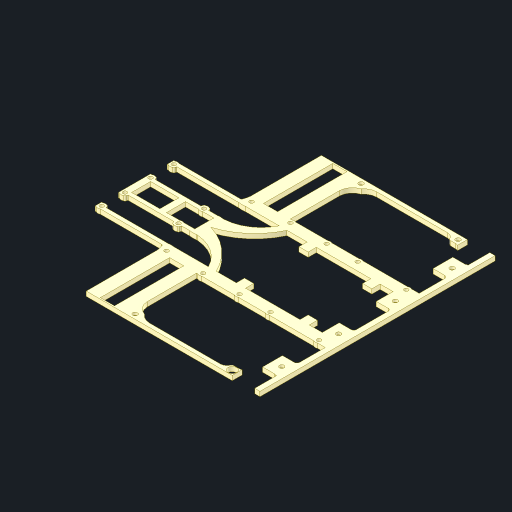
# Autodesk Inventor part: base
Saved by Autodesk Inventor 2023 (Build 270158000, 158)
## iProperties
Created: 2024-05-25
Part Number: base
Material: Nylon 6
Document SubType Name: Modeling
Designer: szymo
Density: 1.12 g/cm^3
Appearance: Nylon 6
Mass: 126.189 g
Surface Area: 671.47 cm^2
Volume: 112.669 cm^3
Author: szymo
Autodesk Inventor part; units mm, degrees
ref_plane "YZ Plane" through (0, 0, 0) normal (1, 0, 0) x (0, 1, 0)
ref_plane "XZ Plane" through (0, 0, 0) normal (0, 1, 0) x (-1, 0, 0)
ref_plane "XY Plane" through (0, 0, 0) normal (0, 0, 1) x (1, 0, 0)
sketch "Sketch1" plane through (0, 0, 0) normal (0, 1, 0) x (-1, 0, 0)
  line L0 (99, 89) -> (-99, 89)
  line L1 (-99, 89) -> (-99, -89)
  line L2 (-99, -89) -> (99, -89)
  line L3 (99, -89) -> (99, 89)
  line L4 (99, 89) -> (-99, -89) construction
  line L5 (-99, 89) -> (99, -89) construction
  line L6 (-85, 89) -> (-85, -89)
  line L7 (-64, 89) -> (-64, 72.5)
  line L8 (-64, 72.5) -> (-81, 72.5)
  line L9 (-81, -72.5) -> (-64, -72.5)
  line L10 (-64, -72.5) -> (-64, -89)
  line L11 (-81, -89) -> (-81, 89)
  point P0 (0, 0)
  dimension "d0" = 198
  dimension "d1" = 178
  dimension "d2" = 14
  dimension "d3" = 16.5
  dimension "d4" = 16.5
  dimension "d9" = 4
  dimension "d10" = 17
  dimension "d11" = 17
  constraints: 24 end point, 8 point on line, 6 perpendicular, 2 horizontal, 2 midpoint, 2 parallel, 1 vertical
  measures "d0" distance of L2.end L1.end
  measures "d1" distance of L1.end L0.end
  measures "d2" distance between parallel lines of L6 L1
  measures "d3" distance between parallel lines of L0 L8
  measures "d4" distance between parallel lines of L9 L2
  measures "d9" distance between parallel lines of L11 L6
  measures "d10" distance between parallel lines of L10 L11
  measures "d11" distance between parallel lines of L11 L7
extrude "Extrusion1" add sketch "Sketch1" along normal blind 3.5 contours L3 L2 L10 L9 L11 L8 L7 L0 | L11 L2 L6 L0
sketch "Sketch2" plane through (0, 0, 0) normal (0, -1, 0) x (1, 0, 0)
  circle A0 centre (77, -64.5) radius 1.2295
  circle A1 centre (77, -21.5) radius 1.2295
  circle A2 centre (77, 21.5) radius 1.2295
  circle A3 centre (77, 64.5) radius 1.2295
  arc A4 (56.6186, 83.1429) -> (58.4256, 82) centre (58.4256, 84) ccw
  line L0 (62, 82) -> (58.4256, 82)
  arc A5 (66.9487, 77.7143) -> (62, 82) centre (62, 77) ccw
  arc A6 (66.9487, 77.7143) -> (68.9282, 76) centre (68.9282, 78) ccw
  line L1 (72.3229, 76) -> (68.9282, 76)
  arc A7 (72.3229, 76) -> (74.3229, 78) centre (72.3229, 78) ccw
  line L2 (74.3229, 81.0104) -> (74.3229, 78)
  arc A8 (79, 86) -> (74.3229, 81.0104) centre (79.3229, 81.0104) ccw
  line L3 (79, 89) -> (79, 86)
  line L4 (-46.5, 89) -> (79, 89)
  line L5 (-46.5, 89) -> (-46.5, 73)
  line L6 (-39.246, 73) -> (-46.5, 73)
  spline S0 degree 3 poles (-38.725, 73.0306) (-38.9029, 73.01) (-39.0786, 73) (-39.246, 73) knots 0 0 0 0 1 1 1 1
  line L7 (-38.725, 88) -> (-38.725, 73.0306)
  line L8 (-24.275, 88) -> (-38.725, 88)
  line L9 (-24.275, 73.0306) -> (-24.275, 88)
  spline S1 degree 3 poles (-23.754, 73) (-23.9214, 73) (-24.0971, 73.01) (-24.275, 73.0306) knots 0 0 0 0 1 1 1 1
  line L10 (-16.5, 73) -> (-23.754, 73)
  arc A9 (-9.5, 82) -> (-16.5, 73) centre (-6.5148, 72.456) ccw
  arc A10 (-1.5, 86) -> (-9.5, 82) centre (-1.5, 76) ccw
  line L11 (52.101, 86) -> (-1.5, 86)
  arc A11 (56.6186, 83.1429) -> (52.101, 86) centre (52.101, 81) ccw
  circle A12 centre (70, 79.5) radius 1.75
  circle A13 centre (-13, 85.5) radius 2.3
  circle A14 centre (60.5017, 85.4375) radius 2.3
  circle A15 centre (70, -82.5) radius 1.75
  arc A16 (58.4256, -82) -> (56.6186, -83.1429) centre (58.4256, -84) ccw
  arc A17 (52.101, -86) -> (56.6186, -83.1429) centre (52.101, -81) ccw
  line L12 (52.101, -86) -> (-1.5, -86)
  arc A18 (-9.5, -82) -> (-1.5, -86) centre (-1.5, -76) ccw
  arc A19 (-16.5, -73) -> (-9.5, -82) centre (-6.5148, -72.456) ccw
  line L13 (-16.5, -73) -> (-23.754, -73)
  spline S2 degree 3 poles (-23.754, -73) (-23.9214, -73) (-24.0971, -73.01) (-24.275, -73.0306) knots 0 0 0 0 1 1 1 1
  line L14 (-24.275, -73.0306) -> (-24.275, -88)
  line L15 (-24.275, -88) -> (-38.725, -88)
  line L16 (-38.725, -88) -> (-38.725, -73.0306)
  spline S3 degree 3 poles (-38.725, -73.0306) (-38.9029, -73.01) (-39.0786, -73) (-39.246, -73) knots 0 0 0 0 1 1 1 1
  line L17 (-39.246, -73) -> (-46.5, -73)
  line L18 (-46.5, -89) -> (-46.5, -73)
  line L19 (-46.5, -89) -> (79, -89)
  line L20 (79, -89) -> (79, -86)
  arc A20 (74.3229, -81.0104) -> (79, -86) centre (79.3229, -81.0104) ccw
  line L21 (74.3229, -81.0104) -> (74.3229, -78)
  arc A21 (74.3229, -78) -> (72.3229, -76) centre (72.3229, -78) ccw
  line L22 (72.3229, -76) -> (68.9282, -76)
  arc A22 (68.9282, -76) -> (66.9487, -77.7143) centre (68.9282, -78) ccw
  arc A23 (62, -82) -> (66.9487, -77.7143) centre (62, -77) ccw
  line L23 (62, -82) -> (58.4256, -82)
  circle A24 centre (-13, -85.5) radius 2.3
  circle A25 centre (60.5017, -85.4375) radius 2.3
  point P0 (0, 0)
  point P1 (-13, -85.5)
  point P2 (-13, 85.5)
  constraints: 6 coincident
hole "m3" at (-13, 0, -85.5) at (60.5017, 0, -85.4375) at (-13, 0, 85.5) at (60.5017, 0, 85.4375) at (77, 0, 64.5) at (77, 0, 21.5) at (77, 0, -21.5) at (77, 0, -64.5) direction (0, 1, 0) diameter 3.6 end through all countersink diameter 6.7 countersink angle 90 clearance for "Countersunk Flat Head Screw ISO 2009/7046" size "M3" standard "ISO"
sketch "Sketch3" plane through (0, 0, 0) normal (0, -1, 0) x (1, 0, 0)
  circle A0 centre (-96.5, -27.3) radius 1.75
  circle A1 centre (-96.5, -9.7) radius 1.75
  circle A2 centre (-96.5, 9.7) radius 1.75
  circle A3 centre (-96.5, 27.3) radius 1.75
  circle A4 centre (-56, 9.7) radius 1.75
  circle A5 centre (-56, -9.7) radius 1.75
  circle A6 centre (-42.5596, -32.1689) radius 1.5
  circle A7 centre (-42.5596, 32.1689) radius 1.75
  circle A8 centre (-13.9698, 33) radius 1.75
  circle A9 centre (13.5198, 33) radius 1.75
  circle A10 centre (37.0073, 33) radius 1.75
  circle A11 centre (73.7355, 33) radius 1.75
  circle A12 centre (73.7355, -33) radius 1.75
  circle A13 centre (37.0073, -33) radius 1.75
  circle A14 centre (-96.5, -27.3) radius 1.75
  circle A15 centre (73.7355, -33) radius 1.75
  circle A16 centre (13.5198, -33) radius 1.75
  circle A17 centre (-42.5596, -32.1689) radius 1.75
  circle A18 centre (-13.9698, -33) radius 1.75
  arc A19 (-94, -25.8) -> (-95, -24.8) centre (-95, -25.8) ccw
  line L0 (-95, -24.8) -> (-99, -24.8)
  line L1 (-99, -29.8) -> (-99, -24.8)
  line L2 (-48.6566, -29.8) -> (-99, -29.8)
  arc A20 (-47.7313, -30.4207) -> (-48.6566, -29.8) centre (-48.6566, -30.8) ccw
  arc A21 (-46.5, -35.5) -> (-47.7313, -30.4207) centre (-63.78, -37) ccw
  line L3 (79, -35.5) -> (-46.5, -35.5)
  line L4 (79, -35.5) -> (79, -30.5)
  line L5 (79, -30.5) -> (-33.3917, -30.5)
  arc A22 (-40.5373, -26.8) -> (-33.3917, -30.5) centre (-33.3917, -21.75) ccw
  line L6 (-40.5373, -26.8) -> (-41.9987, -26.8)
  spline S0 degree 3 poles (-46.8237, -26.8) (-46.5789, -26.8) (-46.2862, -26.7761) (-45.5332, -26.6913) (-44.9243, -26.6) (-44.4112, -26.6) (-43.8981, -26.6) (-43.2892, -26.6913) (-42.5362, -26.7761) (-42.2435, -26.8) (-41.9987, -26.8) knots 0 0 0 0 0.161475 0.161475 0.5 0.5 0.5 0.838525 0.838525 1 1 1 1
  line L7 (-46.8237, -26.8) -> (-94, -26.8)
  line L8 (-94, -26.8) -> (-94, -25.8)
  line L9 (28.681, 30.5) -> (45.3337, 30.5)
  circle A23 centre (37.0073, 33) radius 1.75
  circle A24 centre (-96.5, 27.3) radius 1.75
  circle A25 centre (73.7355, 33) radius 1.75
  circle A26 centre (13.5198, 33) radius 1.75
  circle A27 centre (-42.5596, 32.1689) radius 1.75
  circle A28 centre (-13.9698, 33) radius 1.75
  arc A29 (-95, 24.8) -> (-94, 25.8) centre (-95, 25.8) ccw
  line L10 (-94, 26.8) -> (-94, 25.8)
  line L11 (-46.8237, 26.8) -> (-94, 26.8)
  spline S1 degree 3 poles (-46.8237, 26.8) (-46.5789, 26.8) (-46.2862, 26.7761) (-45.5332, 26.6913) (-44.9243, 26.6) (-44.4112, 26.6) (-43.8981, 26.6) (-43.2892, 26.6913) (-42.5362, 26.7761) (-42.2435, 26.8) (-41.9987, 26.8) knots 0 0 0 0 0.161475 0.161475 0.5 0.5 0.5 0.838525 0.838525 1 1 1 1
  line L12 (-40.5373, 26.8) -> (-41.9987, 26.8)
  arc A30 (-33.3917, 30.5) -> (-40.5373, 26.8) centre (-33.3917, 21.75) ccw
  line L13 (79, 30.5) -> (-33.3917, 30.5)
  line L14 (79, 35.5) -> (79, 30.5)
  line L15 (79, 35.5) -> (-46.5, 35.5)
  arc A31 (-47.7313, 30.4207) -> (-46.5, 35.5) centre (-63.78, 37) ccw
  arc A32 (-48.6566, 29.8) -> (-47.7313, 30.4207) centre (-48.6566, 30.8) ccw
  line L16 (-48.6566, 29.8) -> (-99, 29.8)
  line L17 (-99, 29.8) -> (-99, 24.8)
  line L18 (-95, 24.8) -> (-99, 24.8)
  point P0 (0, 0)
  constraints: 16 coincident
hole "m2.5" at (73.7355, 0, -33) at (37.0073, 0, -33) at (13.5198, 0, -33) at (-13.9698, 0, -33) at (-42.5596, 0, -32.1689) at (73.7355, 0, 33) at (37.0073, 0, 33) at (13.5198, 0, 33) at (-13.9698, 0, 33) at (-42.5596, 0, 32.1689) at (-56, 0, 9.7) at (-56, 0, -9.7) at (-96.5, 0, -9.7) at (-96.5, 0, 9.7) at (-96.5, 0, 27.3) at (-96.5, 0, -27.3) direction (0, 1, 0) diameter 3.1 end through all countersink diameter 5.8 countersink angle 90 clearance for "Countersunk Flat Head Screw ISO 2009/7046" size "M2.5" standard "ISO"
sketch "Sketch4" plane through (0, 0, 0) normal (0, 1, 0) x (1, 0, 0)
  line L0 (-36.8852, -40.5) -> (-31.5, -40.5)
  line L1 (-31.5, -40.5) -> (-26.1148, -40.5)
  line L2 (-26.1148, -40.5) -> (-26.1148, -68.2)
  line L3 (-26.1148, -68.2) -> (-36.8852, -68.2)
  line L4 (-36.8852, -68.2) -> (-36.8852, -40.5)
  line L5 (-26.1148, 40.5) -> (-31.5, 40.5)
  line L6 (-31.5, 40.5) -> (-36.8852, 40.5)
  line L7 (-36.8852, 40.5) -> (-36.8852, 68.2)
  line L8 (-36.8852, 68.2) -> (-26.1148, 68.2)
  line L9 (-26.1148, 68.2) -> (-26.1148, 40.5)
  line L10 (-24.275, 88) -> (-38.725, 88)
  line L11 (-46.5, 89) -> (-46.5, 73)
  line L12 (-46.5, 89) -> (79, 89)
  line L13 (79, 89) -> (79, 86)
  line L14 (74.3229, 81.0104) -> (74.3229, 78)
  line L15 (74.3229, -81.0104) -> (74.3229, -78)
  line L16 (79, -89) -> (79, -86)
  line L17 (-46.5, -89) -> (79, -89)
  line L18 (-46.5, -89) -> (-46.5, -73)
  circle A0 centre (70, -79.5) radius 1.75
  circle A1 centre (37.0073, 33) radius 1.75
  circle A2 centre (-96.5, 27.3) radius 1.75
  circle A3 centre (73.7355, 33) radius 1.75
  circle A4 centre (13.5198, 33) radius 1.75
  circle A5 centre (-42.5596, 32.1689) radius 1.75
  circle A6 centre (-13.9698, 33) radius 1.75
  arc A7 (-95, 24.8) -> (-94, 25.8) centre (-95, 25.8) ccw
  line L19 (-95, 24.8) -> (-99, 24.8)
  line L20 (-99, 29.8) -> (-99, 24.8)
  line L21 (-48.6566, 29.8) -> (-99, 29.8)
  arc A8 (-48.6566, 29.8) -> (-47.7313, 30.4207) centre (-48.6566, 30.8) ccw
  arc A9 (-47.7313, 30.4207) -> (-46.5, 35.5) centre (-63.78, 37) ccw
  line L22 (79, 35.5) -> (-46.5, 35.5)
  line L23 (79, 35.5) -> (79, 30.5)
  line L24 (79, 30.5) -> (-33.3917, 30.5)
  arc A10 (-33.3917, 30.5) -> (-40.5373, 26.8) centre (-33.3917, 21.75) ccw
  line L25 (-40.5373, 26.8) -> (-41.9987, 26.8)
  spline S0 degree 3 poles (-46.8237, 26.8) (-46.5789, 26.8) (-46.2862, 26.7761) (-45.5332, 26.6913) (-44.9243, 26.6) (-44.4112, 26.6) (-43.8981, 26.6) (-43.2892, 26.6913) (-42.5362, 26.7761) (-42.2435, 26.8) (-41.9987, 26.8) knots 0 0 0 0 0.161475 0.161475 0.5 0.5 0.5 0.838525 0.838525 1 1 1 1
  line L26 (-46.8237, 26.8) -> (-94, 26.8)
  line L27 (-94, 26.8) -> (-94, 25.8)
  circle A11 centre (37.0073, -33) radius 1.75
  circle A12 centre (-96.5, -27.3) radius 1.75
  circle A13 centre (73.7355, -33) radius 1.75
  circle A14 centre (13.5198, -33) radius 1.75
  circle A15 centre (-42.5596, -32.1689) radius 1.75
  circle A16 centre (-13.9698, -33) radius 1.75
  arc A17 (-94, -25.8) -> (-95, -24.8) centre (-95, -25.8) ccw
  line L28 (-94, -26.8) -> (-94, -25.8)
  line L29 (-46.8237, -26.8) -> (-94, -26.8)
  spline S1 degree 3 poles (-46.8237, -26.8) (-46.5789, -26.8) (-46.2862, -26.7761) (-45.5332, -26.6913) (-44.9243, -26.6) (-44.4112, -26.6) (-43.8981, -26.6) (-43.2892, -26.6913) (-42.5362, -26.7761) (-42.2435, -26.8) (-41.9987, -26.8) knots 0 0 0 0 0.161475 0.161475 0.5 0.5 0.5 0.838525 0.838525 1 1 1 1
  line L30 (-40.5373, -26.8) -> (-41.9987, -26.8)
  arc A18 (-40.5373, -26.8) -> (-33.3917, -30.5) centre (-33.3917, -21.75) ccw
  line L31 (79, -30.5) -> (-33.3917, -30.5)
  line L32 (79, -35.5) -> (79, -30.5)
  line L33 (79, -35.5) -> (-46.5, -35.5)
  arc A19 (-46.5, -35.5) -> (-47.7313, -30.4207) centre (-63.78, -37) ccw
  arc A20 (-47.7313, -30.4207) -> (-48.6566, -29.8) centre (-48.6566, -30.8) ccw
  line L34 (-48.6566, -29.8) -> (-99, -29.8)
  line L35 (-99, -29.8) -> (-99, -24.8)
  line L36 (-95, -24.8) -> (-99, -24.8)
  line L37 (44.7969, 39.7458) -> (-15.2031, 39.7458) construction
  line L38 (-15.2031, 39.7458) -> (-15.2031, 69.7458) construction
  line L39 (44.7969, 69.7458) -> (-15.2031, 69.7458) construction
  line L40 (44.7969, 39.7458) -> (44.7969, 69.7458) construction
  line L41 (44.5627, -68.989) -> (-15.4373, -68.989) construction
  line L42 (-15.4373, -68.989) -> (-15.4373, -38.989) construction
  line L43 (44.5627, -38.989) -> (-15.4373, -38.989) construction
  line L44 (44.5627, -68.989) -> (44.5627, -38.989) construction
  line L45 (85, 89) -> (99, 89)
  line L46 (99, 89) -> (99, -89)
  line L47 (85, -89) -> (99, -89)
  line L48 (85, 89) -> (85, -89)
  circle A21 centre (77, -21.5) radius 1.2295
  circle A22 centre (77, 64.5) radius 1.2295
  circle A23 centre (77, 21.5) radius 1.2295
  circle A24 centre (77, -64.5) radius 1.2295
  line L49 (70, 72) -> (79, 72)
  arc A25 (79, 72) -> (81, 74) centre (79, 74) ccw
  line L50 (81, 74) -> (81, 89)
  line L51 (81, 89) -> (85, 89)
  line L52 (85, 89) -> (85, -89)
  line L53 (81, -89) -> (85, -89)
  line L54 (81, -89) -> (81, -74)
  arc A26 (81, -74) -> (79, -72) centre (79, -74) ccw
  line L55 (79, -72) -> (70, -72)
  line L56 (70, -57) -> (70, -72)
  line L57 (70, -57) -> (79, -57)
  arc A27 (79, -57) -> (81, -55) centre (79, -55) ccw
  line L58 (81, -55) -> (81, -31)
  arc A28 (81, -31) -> (79, -29) centre (79, -31) ccw
  line L59 (79, -29) -> (70, -29)
  line L60 (70, -14) -> (70, -29)
  line L61 (70, -14) -> (79, -14)
  arc A29 (79, -14) -> (81, -12) centre (79, -12) ccw
  line L62 (81, -12) -> (81, 12)
  arc A30 (81, 12) -> (79, 14) centre (79, 12) ccw
  line L63 (79, 14) -> (70, 14)
  line L64 (70, 29) -> (70, 14)
  line L65 (70, 29) -> (79, 29)
  arc A31 (79, 29) -> (81, 31) centre (79, 31) ccw
  line L66 (81, 31) -> (81, 55)
  arc A32 (81, 55) -> (79, 57) centre (79, 55) ccw
  line L67 (79, 57) -> (70, 57)
  line L68 (70, 72) -> (70, 57)
  line L69 (60, -27.5) -> (5, -27.5)
  line L70 (5, -27.5) -> (5, 27.5)
  line L71 (5, 27.5) -> (60, 27.5)
  line L72 (60, 27.5) -> (60, -27.5)
  circle A33 centre (56.6, -24.1) radius 1.6
  circle A34 centre (8.4, -24.1) radius 1.6
  circle A35 centre (56.6, 24.1) radius 1.6
  circle A36 centre (8.4, 24.1) radius 1.6
  line L73 (-99, -7) -> (-37.5, -7) construction
  line L74 (-99, 7) -> (-99, -7) construction
  line L75 (-37.5, 7) -> (-99, 7) construction
  line L76 (-37.5, -7) -> (-37.5, 7) construction
  circle A37 centre (-56, 9.7) radius 1.75
  circle A38 centre (-96.5, 9.7) radius 1.75
  arc A39 (-57.5, 12.2) -> (-58.5, 11.2) centre (-57.5, 11.2) ccw
  line L77 (-57.5, 12.2) -> (-54.5, 12.2)
  arc A40 (-53.5, 11.2) -> (-54.5, 12.2) centre (-54.5, 11.2) ccw
  line L78 (-53.5, 11.2) -> (-53.5, 10.2)
  line L79 (-53.5, 10.2) -> (-46.8237, 10.2)
  spline S2 degree 3 poles (-41.9987, 10.2) (-42.2435, 10.2) (-42.5362, 10.2239) (-43.2892, 10.3087) (-43.8981, 10.4) (-44.4112, 10.4) (-44.9243, 10.4) (-45.5332, 10.3087) (-46.2862, 10.2239) (-46.5789, 10.2) (-46.8237, 10.2) knots 0 0 0 0 0.161475 0.161475 0.5 0.5 0.5 0.838525 0.838525 1 1 1 1
  line L80 (-41.9987, 10.2) -> (-41.148, 10.2)
  line L81 (-41.148, 10.2) -> (-41.148, 7.2)
  line L82 (-41.148, 7.2) -> (-99, 7.2)
  line L83 (-99, 7.2) -> (-99, 12.2)
  line L84 (-99, 12.2) -> (-95, 12.2)
  arc A41 (-94, 11.2) -> (-95, 12.2) centre (-95, 11.2) ccw
  line L85 (-94, 10.2) -> (-94, 11.2)
  line L86 (-94, 10.2) -> (-58.5, 10.2)
  line L87 (-58.5, 10.2) -> (-58.5, 11.2)
  circle A42 centre (-56, -9.7) radius 1.75
  circle A43 centre (-96.5, -9.7) radius 1.75
  arc A44 (-58.5, -11.2) -> (-57.5, -12.2) centre (-57.5, -11.2) ccw
  line L88 (-58.5, -10.2) -> (-58.5, -11.2)
  line L89 (-94, -10.2) -> (-58.5, -10.2)
  line L90 (-94, -10.2) -> (-94, -11.2)
  arc A45 (-95, -12.2) -> (-94, -11.2) centre (-95, -11.2) ccw
  line L91 (-99, -12.2) -> (-95, -12.2)
  line L92 (-99, -7.2) -> (-99, -12.2)
  line L93 (-41.148, -7.2) -> (-99, -7.2)
  line L94 (-41.148, -10.2) -> (-41.148, -7.2)
  line L95 (-41.9987, -10.2) -> (-41.148, -10.2)
  spline S3 degree 3 poles (-41.9987, -10.2) (-42.2435, -10.2) (-42.5362, -10.2239) (-43.2892, -10.3087) (-43.8981, -10.4) (-44.4112, -10.4) (-44.9243, -10.4) (-45.5332, -10.3087) (-46.2862, -10.2239) (-46.5789, -10.2) (-46.8237, -10.2) knots 0 0 0 0 0.161475 0.161475 0.5 0.5 0.5 0.838525 0.838525 1 1 1 1
  line L96 (-53.5, -10.2) -> (-46.8237, -10.2)
  line L97 (-53.5, -11.2) -> (-53.5, -10.2)
  arc A46 (-54.5, -12.2) -> (-53.5, -11.2) centre (-54.5, -11.2) ccw
  line L98 (-57.5, -12.2) -> (-54.5, -12.2)
  line L99 (81, 35.5) -> (-46.5, 35.5)
  line L100 (-46.5, 35.5) -> (-46.5, 29.8)
  line L101 (-46.5, 29.8) -> (-99, 29.8)
  line L102 (-99, 29.8) -> (-99, 24.8)
  line L103 (-99, 24.8) -> (-95, 24.8)
  line L104 (-94, 25.8) -> (-94, 26.8)
  line L105 (-94, 26.8) -> (-40.5373, 26.8)
  line L106 (-40.5373, 26.8) -> (70, 26.8)
  line L107 (81, -35.5) -> (-46.5, -35.5)
  line L108 (-46.5, -35.5) -> (-46.5, -29.8)
  line L109 (-46.5, -29.8) -> (-99, -29.8)
  line L110 (-99, -24.8) -> (-99, -29.8)
  line L111 (-99, -24.8) -> (-95, -24.8)
  line L112 (-94, -25.8) -> (-94, -26.8)
  line L113 (-94, -26.8) -> (-40.5373, -26.8)
  line L114 (-40.5373, -26.8) -> (70, -26.8)
  line L115 (60.1, 27.6) -> (53.1, 27.6)
  line L116 (53.1, 27.6) -> (53.1, 20.6)
  line L117 (53.1, 20.6) -> (60.1, 20.6)
  line L118 (60.1, 20.6) -> (60.1, 27.6)
  line L119 (60.1, 27.6) -> (53.1, 20.6) construction
  line L120 (53.1, 27.6) -> (60.1, 20.6) construction
  line L121 (60.1, -20.6) -> (53.1, -20.6)
  line L122 (53.1, -20.6) -> (53.1, -27.6)
  line L123 (53.1, -27.6) -> (60.1, -27.6)
  line L124 (60.1, -27.6) -> (60.1, -20.6)
  line L125 (60.1, -20.6) -> (53.1, -27.6) construction
  line L126 (53.1, -20.6) -> (60.1, -27.6) construction
  line L127 (11.9, -20.6) -> (4.9, -20.6)
  line L128 (4.9, -20.6) -> (4.9, -27.6)
  line L129 (4.9, -27.6) -> (11.9, -27.6)
  line L130 (11.9, -27.6) -> (11.9, -20.6)
  line L131 (11.9, -20.6) -> (4.9, -27.6) construction
  line L132 (4.9, -20.6) -> (11.9, -27.6) construction
  line L133 (11.9, 27.6) -> (4.9, 27.6)
  line L134 (4.9, 27.6) -> (4.9, 20.6)
  line L135 (4.9, 20.6) -> (11.9, 20.6)
  line L136 (11.9, 20.6) -> (11.9, 27.6)
  line L137 (11.9, 27.6) -> (4.9, 20.6) construction
  line L138 (4.9, 27.6) -> (11.9, 20.6) construction
  line L139 (-99, 7.2) -> (-94, 7.2)
  line L140 (-94, 7.2) -> (-94, -7.2)
  line L141 (-94, -7.2) -> (-99, -7.2)
  line L142 (-99, -7.2) -> (-99, 7.2)
  line L143 (-41.148, 7.2) -> (-46.148, 7.2)
  line L144 (-46.148, 7.2) -> (-46.148, -7.2)
  line L145 (-46.148, -7.2) -> (-41.148, -7.2)
  line L146 (-41.148, -7.2) -> (-41.148, 7.2)
  line L147 (-72.574, 7.2) -> (-67.574, 7.2)
  line L148 (-67.574, 7.2) -> (-67.574, -7.2)
  line L149 (-67.574, -7.2) -> (-72.574, -7.2)
  line L150 (-72.574, -7.2) -> (-72.574, 7.2)
  arc A47 (-41.148, 10.2) -> (-13.9698, 33) centre (-43.1088, 40.1359) ccw
  arc A48 (-13.9698, -33) -> (-41.148, -10.2) centre (-43.1088, -40.1359) ccw
  line L151 (-13.9698, 33) -> (-7.9698, 33)
  line L152 (-13.9698, -33) -> (-7.9698, -33)
  arc A49 (-41.148, 0) -> (-7.9698, 33) centre (-55.7201, 47.8294) ccw
  arc A50 (-7.9698, -33) -> (-41.148, 0) centre (-55.7201, -47.8294) ccw
  line L153 (-36.8852, 35.5) -> (-46.5, 35.5)
  line L154 (-46.5, 35.5) -> (-46.5, 89)
  line L155 (-46.5, 89) -> (-36.8852, 89)
  line L156 (-36.8852, 89) -> (-36.8852, 35.5)
  line L157 (-26.1148, 35.5) -> (-16.5, 35.5)
  line L158 (-16.5, 35.5) -> (-16.5, 89)
  line L159 (-16.5, 89) -> (-26.1148, 89)
  line L160 (-26.1148, 89) -> (-26.1148, 35.5)
  line L161 (-46.5, -35.5) -> (-36.8852, -35.5)
  line L162 (-36.8852, -35.5) -> (-36.8852, -89)
  line L163 (-36.8852, -89) -> (-46.5, -89)
  line L164 (-46.5, -89) -> (-46.5, -35.5)
  line L165 (-26.1148, -89) -> (-16.5, -89)
  line L166 (-16.5, -89) -> (-16.5, -35.5)
  line L167 (-16.5, -35.5) -> (-26.1148, -35.5)
  line L168 (-26.1148, -35.5) -> (-26.1148, -89)
  arc A51 (-99, -28.7697) -> (-99, -25.8303) centre (-96.5, -27.3) ccw
  line L169 (-99, -11.1697) -> (-99, -25.8303)
  arc A52 (-99, -11.1697) -> (-99, -8.2303) centre (-96.5, -9.7) ccw
  line L170 (-99, 8.2303) -> (-99, -8.2303)
  arc A53 (-99, 8.2303) -> (-99, 11.1697) centre (-96.5, 9.7) ccw
  line L171 (-99, 25.8303) -> (-99, 11.1697)
  arc A54 (-99, 25.8303) -> (-99, 28.7697) centre (-96.5, 27.3) ccw
  line L172 (-99, 89) -> (-99, 28.7697)
  line L173 (64, 89) -> (-99, 89)
  line L174 (64, 72.5) -> (64, 89)
  circle A55 centre (60.5017, 85.4375) radius 3.35
  line L175 (81, 72.5) -> (64, 72.5)
  line L176 (81, 89) -> (81, 72.5)
  line L177 (85, 89) -> (81, 89)
  line L178 (85, -89) -> (85, 89)
  line L179 (81, -89) -> (85, -89)
  line L180 (81, -72.5) -> (81, -89)
  line L181 (64, -72.5) -> (81, -72.5)
  line L182 (64, -89) -> (64, -72.5)
  circle A56 centre (60.5017, -85.4375) radius 3.35
  line L183 (-99, -89) -> (64, -89)
  line L184 (-99, -28.7697) -> (-99, -89)
  circle A57 centre (-56, -9.7) radius 2.9
  circle A58 centre (-13.9698, -33) radius 2.9
  circle A59 centre (37.0073, -33) radius 2.9
  circle A60 centre (-42.5596, 32.1689) radius 2.9
  circle A61 centre (13.5198, 33) radius 2.9
  circle A62 centre (73.7355, 33) radius 2.9
  circle A63 centre (37.0073, 33) radius 2.9
  circle A64 centre (-13.9698, 33) radius 2.9
  circle A65 centre (73.7355, -33) radius 2.9
  circle A66 centre (13.5198, -33) radius 2.9
  circle A67 centre (-42.5596, -32.1689) radius 2.9
  circle A68 centre (-56, 9.7) radius 2.9
  circle A69 centre (77, 64.5) radius 3.35
  circle A70 centre (77, -21.5) radius 3.35
  circle A71 centre (-13, 85.5) radius 3.35
  circle A72 centre (-13, -85.5) radius 3.35
  circle A73 centre (77, -64.5) radius 3.35
  circle A74 centre (77, 21.5) radius 3.35
  line L185 (52.101, -86) -> (-1.5, -86)
  line L186 (72.3229, -76) -> (68.9282, -76)
  arc A75 (58.4256, -82) -> (56.6186, -83.1429) centre (58.4256, -84) ccw
  line L187 (62, -82) -> (58.4256, -82)
  arc A76 (62, -82) -> (66.9487, -77.7143) centre (62, -77) ccw
  arc A77 (68.9282, -76) -> (66.9487, -77.7143) centre (68.9282, -78) ccw
  arc A78 (74.3229, -78) -> (72.3229, -76) centre (72.3229, -78) ccw
  arc A79 (74.3229, -81.0104) -> (79, -86) centre (79.3229, -81.0104) ccw
  line L188 (-39.246, -73) -> (-46.5, -73)
  spline S4 degree 3 poles (-38.725, -73.0306) (-38.9029, -73.01) (-39.0786, -73) (-39.246, -73) knots 0 0 0 0 1 1 1 1
  line L189 (-38.725, -88) -> (-38.725, -73.0306)
  line L190 (-24.275, -88) -> (-38.725, -88)
  line L191 (-24.275, -73.0306) -> (-24.275, -88)
  spline S5 degree 3 poles (-23.754, -73) (-23.9214, -73) (-24.0971, -73.01) (-24.275, -73.0306) knots 0 0 0 0 1 1 1 1
  line L192 (-16.5, -73) -> (-23.754, -73)
  arc A80 (-16.5, -73) -> (-9.5, -82) centre (-6.5148, -72.456) ccw
  arc A81 (-9.5, -82) -> (-1.5, -86) centre (-1.5, -76) ccw
  arc A82 (52.101, -86) -> (56.6186, -83.1429) centre (52.101, -81) ccw
  circle A83 centre (60.5017, -85.4375) radius 2.3
  arc A84 (56.6186, 83.1429) -> (58.4256, 82) centre (58.4256, 84) ccw
  arc A85 (56.6186, 83.1429) -> (52.101, 86) centre (52.101, 81) ccw
  line L193 (52.101, 86) -> (-1.5, 86)
  arc A86 (-1.5, 86) -> (-9.5, 82) centre (-1.5, 76) ccw
  arc A87 (-9.5, 82) -> (-16.5, 73) centre (-6.5148, 72.456) ccw
  line L194 (-16.5, 73) -> (-23.754, 73)
  spline S6 degree 3 poles (-23.754, 73) (-23.9214, 73) (-24.0971, 73.01) (-24.275, 73.0306) knots 0 0 0 0 1 1 1 1
  line L195 (-24.275, 73.0306) -> (-24.275, 88)
  line L196 (-38.725, 88) -> (-38.725, 73.0306)
  spline S7 degree 3 poles (-38.725, 73.0306) (-38.9029, 73.01) (-39.0786, 73) (-39.246, 73) knots 0 0 0 0 1 1 1 1
  line L197 (-39.246, 73) -> (-46.5, 73)
  arc A88 (79, 86) -> (74.3229, 81.0104) centre (79.3229, 81.0104) ccw
  arc A89 (72.3229, 76) -> (74.3229, 78) centre (72.3229, 78) ccw
  line L198 (72.3229, 76) -> (68.9282, 76)
  arc A90 (66.9487, 77.7143) -> (68.9282, 76) centre (68.9282, 78) ccw
  arc A91 (66.9487, 77.7143) -> (62, 82) centre (62, 77) ccw
  line L199 (62, 82) -> (58.4256, 82)
  circle A92 centre (60.5017, 85.4375) radius 2.3
  circle A93 centre (-13, -85.5) radius 2.3
  circle A94 centre (70, 82.5) radius 1.75
  circle A95 centre (-13, 85.5) radius 2.3
  point P0 (0, 0)
  point P1 (-24.275, 74)
  point P2 (-38.725, 74)
  point P3 (69, 76)
  point P4 (69, -76)
  point P5 (-38.725, -74)
  point P6 (-24.275, -74)
  point P7 (11.9, 26.8)
  point P8 (4.9, 26.8)
  point P9 (-10.3575, 26.8)
  point P10 (-10.3575, -26.8)
  point P11 (4.9, -26.8)
  point P12 (11.9, -26.8)
  point P13 (53.1, -26.8)
  point P14 (60.1, -26.8)
  point P15 (60.1, 26.8)
  point P16 (53.1, 26.8)
  point P17 (58, -83.3124)
  point P18 (58, -81.6876)
  point P19 (80.3229, -72.5)
  point P20 (75.2052, -35.5)
  point P21 (72.2658, -35.5)
  point P22 (38.477, -35.5)
  point P23 (35.5376, -35.5)
  point P24 (14.9895, -35.5)
  point P25 (12.0501, -35.5)
  point P26 (-12.5001, -35.5)
  point P27 (-15.4395, -35.5)
  point P28 (-15.4395, 35.5)
  point P29 (-12.5001, 35.5)
  point P30 (12.0501, 35.5)
  point P31 (14.9895, 35.5)
  point P32 (35.5376, 35.5)
  point P33 (38.477, 35.5)
  point P34 (72.2658, 35.5)
  point P35 (75.2052, 35.5)
  point P36 (80.3229, 72.5)
  point P37 (58, 81.6876)
  point P38 (58, 83.3124)
  point P39 (-95.0303, -29.8)
  point P40 (-97.9697, -29.8)
  point P41 (-46.5, -73)
  point P42 (-46.5, 35.5)
  point P43 (-97.9697, 29.8)
  point P44 (-95.0303, 29.8)
  point P45 (-26.1148, 88)
  point P46 (-36.8852, 88)
  point P47 (-94, -25.8303)
  point P48 (-93.6434, -26.8)
  point P49 (-16.2358, -26.8)
  point P50 (-53.1434, -10.2)
  point P51 (-53.5, -11.1697)
  point P52 (-54.5303, -12.2)
  point P53 (-57.4697, -12.2)
  point P54 (-58.5, -11.1697)
  point P55 (-58.8566, -10.2)
  point P56 (-93.6434, -10.2)
  point P57 (-94, -11.1697)
  point P58 (-95.0303, -12.2)
  point P59 (-97.9697, -12.2)
  point P60 (-97.9697, -24.8)
  point P61 (-95.0303, -24.8)
  point P62 (-95.0303, 24.8)
  point P63 (-97.9697, 24.8)
  point P64 (-97.9697, 12.2)
  point P65 (-95.0303, 12.2)
  point P66 (-94, 11.1697)
  point P67 (-93.6434, 10.2)
  point P68 (-58.8566, 10.2)
  point P69 (-58.5, 11.1697)
  point P70 (-57.4697, 12.2)
  point P71 (-54.5303, 12.2)
  point P72 (-53.5, 11.1697)
  point P73 (-53.1434, 10.2)
  point P74 (-16.2358, 26.8)
  point P75 (-93.6434, 26.8)
  point P76 (-94, 25.8303)
  point P77 (-54.5303, 7.2)
  point P78 (-57.4697, 7.2)
  point P79 (-57.4697, -7.2)
  point P80 (-54.5303, -7.2)
  point P81 (-26.1148, -88)
  point P82 (57.9287, -82.0627)
  point P83 (75.2052, -35.5)
  point P84 (72.2658, -35.5)
  point P85 (38.477, -35.5)
  point P86 (35.5376, -35.5)
  point P87 (14.9895, -35.5)
  point P88 (12.0501, -35.5)
  point P89 (-12.5001, -35.5)
  point P90 (-15.4395, -35.5)
  point P91 (-99, -25.8303)
  point P92 (-99, -28.7697)
  point P93 (70.9014, 81)
  point P94 (69.0986, 81)
  point P95 (57.9287, 82.0627)
  point P96 (-15.4395, 35.5)
  point P97 (-12.5001, 35.5)
  point P98 (12.0501, 35.5)
  point P99 (14.9895, 35.5)
  point P100 (35.5376, 35.5)
  point P101 (38.477, 35.5)
  point P102 (72.2658, 35.5)
  point P103 (75.2052, 35.5)
  point P104 (-99, 28.7697)
  point P105 (-99, 25.8303)
  point P106 (-93.6434, -26.8)
  point P107 (-94, -25.8303)
  point P108 (-94, 25.8303)
  point P109 (-95.0303, 24.8)
  point P110 (-93.6434, 26.8)
  point P111 (-97.9697, 24.8)
  point P112 (-36.8852, -88)
  point P113 (64, -81.5826)
  point P114 (64, 81.5826)
  point P115 (-46.5, 35.5)
  dimension "d26" = 7
  dimension "d27" = 7
  dimension "d28" = 7
  dimension "d29" = 7
  dimension "d30" = 7
  dimension "d31" = 7
  dimension "d32" = 7
  dimension "d33" = 7
  dimension "d34" = 5
  dimension "d35" = 5
  dimension "d36" = 5
  dimension "d37" = 21.426
  dimension "d38" = 21.426
  dimension "d39" = 30
  dimension "d40" = 30
  dimension "d41" = 6
  dimension "d42" = 6
  dimension "d43" = 50
  dimension "d44" = 50
  constraints: 160 end point, 22 parallel, 19 horizontal, 18 point on line, 16 perpendicular, 9 collinear, 9 midpoint, 8 point on circle, 5 vertical, 4 centre point, 1 tangent, 10 other
  measures "d26" distance of L117.end L116.end
  measures "d27" distance of L116.end L115.end
  measures "d28" distance of L123.end L122.end
  measures "d29" distance of L122.end L121.end
  measures "d30" distance of L129.end L128.end
  measures "d31" distance of L128.end L127.end
  measures "d32" distance of L135.end L134.end
  measures "d33" distance of L134.end L133.end
  measures "d34" distance of L140.end L141.end
  measures "d35" distance of L145.end L144.end
  measures "d36" distance of L148.end L149.end
  measures "d37" distance between parallel lines of L150 L140
  measures "d38" distance between parallel lines of L144 L148
  measures "d39" radius of A47
  measures "d40" radius of A48
  measures "d41" distance of L151.start L151.end
  measures "d42" distance of L152.start L152.end
  measures "d43" radius of A49
  measures "d44" radius of A50
extrude "zeberka" cut sketch "Sketch4" along normal blind 3.5 contours L162 L33 L168 L1 L0 | L0 L1 L2 L3 L4 | L3 L168 L190 L162 | L164 L18 L183 L184 L34 A51 A20 A19 | L33 A58 A66 A59 A65 L107 L58 A27 L57 L56 L55 A26 L181 L182 A76 L187 A75 A82 L185 A81 A80 L166 | A51 L28 A17 L36 L169 L91 A52 A45 L90 L89 A57 L88 A44 L98 A46 L97 L96 S3 L95 A48 L114 L30 S1 L29 | A50 A49 L106 L134 L135 L70 L127 L128 L114 | L181 L180 A26 | L93 A57 L148 L82 A68 L144 | L70 L135 L136 L106 L116 L117 L72 L121 L122 L114 L130 L127 | L80 S2 L79 A68 L78 A40 L77 A39 L87 L86 A53 L85 A41 L84 L171 L19 A54 A7 L27 L26 S0 L25 L106 A47 | L22 A64 L158 A87 A86 L193 A85 A84 L199 A91 L174 L175 A25 L49 L68 L67 A32 L66 L99 A62 A63 A61 | L72 L117 L118 L106 L64 L63 A30 L62 A29 L61 L60 L114 L124 L121 | L93 L140 L82 L150 | L176 L175 A25 | A54 L21 L172 L173 L11 L154 A9 A8 | L22 L156 L6 L5 L160 | L5 L6 L7 L8 L9 | L8 L156 L10 L160 | A56 | A83
equation "\"d37\" = d38"
body "Solid1"
